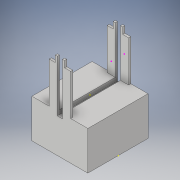
# Autodesk Inventor part: Suporte_motor
Saved by Autodesk Inventor 2018 (Build 220112000, 112)
## iProperties
Created: 2018-02-28
Part Number: Suporte_motor
Material: Generic
Document SubType Name: Modeling
Designer: matheus
Density: 1 g/cm^3
Appearance: Default
Author: matheus
Autodesk Inventor part; units mm, degrees
ref_plane "YZ Plane" through (0, 0, 0) normal (1, 0, 0) x (0, 1, 0)
ref_plane "XZ Plane" through (0, 0, 0) normal (0, 1, 0) x (-1, 0, 0)
ref_plane "XY Plane" through (0, 0, 0) normal (0, 0, 1) x (1, 0, 0)
sketch "Sketch1" plane through (0, 0, 0) normal (0, 1, 0) x (-1, 0, 0)
  point P0 (0, 0)
sketch "Sketch2" plane through (0, 0, 0) normal (0, 1, 0) x (-1, 0, 0)
  line L0 (-13, 14) -> (13, 14)
  line L1 (13, 14) -> (13, -14)
  line L2 (13, -14) -> (-13, -14)
  line L3 (-13, -14) -> (-13, 14)
  line L4 (-13, 14) -> (13, -14) construction
  line L5 (13, 14) -> (-13, -14) construction
  point P0 (0, 0)
  dimension "d0" = 26
  dimension "d1" = 28
  constraints: 12 end point, 2 midpoint, 2 parallel, 1 horizontal, 1 perpendicular
  measures "d0" distance of L1.end L2.end
  measures "d1" distance of L0.end L1.end
extrude "Extrusion1" add sketch "Sketch2" along normal blind 18
sketch "Sketch5" plane through (13, 0, 14) normal (1, 0, 0) x (0, 0, -1)
  point P0 (14, 0)
  point P1 (17, 39.5)
  point P2 (11, 39.5)
sketch "Sketch7" plane through (0, 18, 0) normal (0, 1, 0) x (1, 0, 0)
  point P0 (0, 0)
sketch "Sketch8" plane through (0, 18, 0) normal (0, 1, 0) x (1, 0, 0)
  line L0 (13, 14) -> (-13, 14) projected
  line L1 (13, 14) -> (5, 14)
  line L2 (-5, 14) -> (-4, 14)
  line L3 (-5, 14) -> (5, 14)
  line L4 (5, 14) -> (5, 13)
  line L5 (5, 13) -> (-5, 13)
  line L6 (-5, 13) -> (-5, 14)
  line L7 (-13, -14) -> (13, -14) projected
  line L8 (-5, -14) -> (5, -14)
  line L9 (5, -14) -> (5, -13)
  line L10 (5, -13) -> (-5, -13)
  line L11 (-5, -13) -> (-5, -14)
  point P0 (0, 0)
  dimension "d22" = 8
  dimension "d23" = 8
  dimension "d24" = 1
  dimension "d26" = 10
  dimension "d27" = 1
  constraints: 20 end point, 5 point on line, 4 parallel, 2 horizontal, 2 perpendicular
  measures "d22" distance of L0.end L2.start
  measures "d23" distance of L0.start L1.end
  measures "d24" distance of L2.start L2.end
  measures "d26" distance of L10.end L9.end
  measures "d27" distance of L9.end L8.end
extrude "Extrusion5" add sketch "Sketch8" along normal blind 22
sketch "Sketch9" plane through (-13, 0, 14) normal (0, 0, 1) x (1, 0, 0)
  line L0 (8, 40) -> (18, 40) projected
  line L1 (10.7548, 39.8791) -> (11.7548, 39.8791) construction
  line L2 (11.7548, 15.8791) -> (14.1548, 15.8791)
  line L3 (14.1548, 15.8791) -> (14.1548, 40)
  line L4 (11.7548, 15.8791) -> (11.7548, 39.8791)
  line L5 (8, 40) -> (10.8, 40)
  line L6 (10.8, 40) -> (10.8, 37)
  line L7 (10.8, 37) -> (8, 37)
  line L8 (8, 37) -> (8, 40)
  line L9 (18, 40) -> (15.2, 40)
  line L10 (15.2, 40) -> (15.2, 37)
  line L11 (15.2, 37) -> (18, 37)
  line L12 (18, 37) -> (18, 40)
  point P0 (13, 0)
  dimension "d38" = 2.4
  dimension "d39" = 2.8
  dimension "d40" = 3
  dimension "d41" = 2.8
  constraints: 24 end point, 4 parallel, 3 horizontal, 3 perpendicular, 2 point on line, 1 vertical
  measures "d38" distance of L2.start L2.end
  measures "d39" distance of L6.end L7.end
  measures "d40" distance of L5.end L6.end
  measures "d41" distance of L11.end L10.end
extrude "Extrusion6" cut sketch "Sketch9" along normal mid plane 100
sketch "Sketch10" plane through (-13, 0, 14) normal (0, 0, 1) x (1, 0, 0)
  line L0 (10.8, 40) -> (10.8, 37) projected
  line L1 (11.8, 40) -> (11.8, 16)
  line L2 (11.8, 16) -> (14.2, 16)
  line L3 (14.2, 16) -> (14.2, 40)
  line L4 (11.8, 40) -> (14.2, 40)
  line L5 (15.2, 40) -> (10.8, 40) projected
  point P0 (13, 0)
  dimension "d44" = 1
  dimension "d45" = 24
  dimension "d46" = 2.4
  constraints: 8 end point, 2 perpendicular, 1 collinear
  measures "d44" distance of L0.start L1.start
  measures "d45" distance of L1.start L1.end
  measures "d46" distance of L1.end L2.end
extrude "Extrusion7" cut sketch "Sketch10" along normal mid plane 100
body "Solid1"
